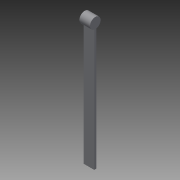
# Autodesk Inventor part: Part1
Saved by Autodesk Inventor 2013 (Build 170138000, 138)
## iProperties
Created: 2013-08-06
Part Number: Part1
Material: 一般
Document SubType Name: Modeling
Designer: victor
Density: 1 g/cm^3
Author: victor
Autodesk Inventor part; units mm, degrees
ref_plane "YZ Plane" through (0, 0, 0) normal (1, 0, 0) x (0, 1, 0)
ref_plane "XZ Plane" through (0, 0, 0) normal (0, 1, 0) x (-1, 0, 0)
ref_plane "XY Plane" through (0, 0, 0) normal (0, 0, 1) x (1, 0, 0)
sketch "スケッチ1" plane through (0, 0, 0) normal (1, 0, 0) x (0, 1, 0)
  line L0 (-7.7246, 3.6677) -> (-2.7246, 3.6677)
  line L1 (-2.7246, 3.6677) -> (-2.7246, -58.3323)
  line L2 (-2.7246, -58.3323) -> (-7.7246, -58.3323)
  line L3 (-7.7246, -58.3323) -> (-7.7246, 3.6677)
  point P0 (0, 0)
  dimension "d0" = 5
  dimension "d2" = 62
  constraints: 8 end point, 2 parallel, 1 horizontal, 1 perpendicular
  measures "d0" distance of L0.start L0.end
  measures "d2" distance of L0.end L1.end
extrude "押し出し1" add sketch "スケッチ1" along normal blind 5
sketch "スケッチ2" plane through (0, 0, 0) normal (-1, 0, 0) x (0, 0, 1)
  line L0 (3.6677, -7.7246) -> (3.6677, -2.7246) projected
  line L1 (3.6677, -2.7246) -> (-58.3323, -2.7246) projected
  line L2 (-58.3323, -2.7246) -> (-58.3323, -7.7246) projected
  line L3 (-58.3323, -7.7246) -> (3.6677, -7.7246) projected
  line L4 (-1.3323, -4.7246) -> (-58.3323, -4.7246)
  line L5 (-58.3323, -4.7246) -> (-58.3323, -5.7246)
  line L6 (-58.3323, -5.7246) -> (-1.3323, -5.7246)
  arc A0 (-1.2818, -5.7246) -> (-1.2818, -4.7246) centre (1.1677, -5.2246) ccw
  line L7 (-1.3323, -5.7246) -> (-1.2818, -5.7246)
  line L8 (-1.3323, -4.7246) -> (-1.2818, -4.7246)
  point P0 (0, 0)
  dimension "d5" = 1
  dimension "d7" = 2
  dimension "d9" = 5
  constraints: 10 end point, 2 parallel, 2 point on circle, 1 centre point, 1 horizontal, 1 perpendicular, 1 point on line, 1 tangent
  measures "d5" distance of L4.end L5.end
  measures "d7" distance between parallel lines of L3 L6
  measures "d9" diameter of A0
extrude "押し出し2" cut sketch "スケッチ2" against normal blind 5 contours L3 A0 L0 | A0 L1 L0 | L3 L2 L6 L7 A0 | A0 L8 L4 L2 L1
